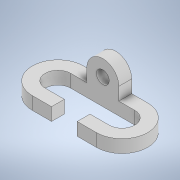
# Autodesk Inventor part: Assignment 3.4 - Coupling Base
Saved by Autodesk Inventor 2022 (Build 260153000, 153)
## iProperties
Created: 2021-05-23
Part Number: Assignment 3.4 - Coupling Base
Material: Generic
Document SubType Name: Modeling
Designer: Aaron
Density: 1 g/cm^3
Appearance: Default
Author: Aaron
Autodesk Inventor part; units mm, degrees
ref_plane "YZ Plane" through (0, 0, 0) normal (1, 0, 0) x (0, 1, 0)
ref_plane "XZ Plane" through (0, 0, 0) normal (0, 1, 0) x (-1, 0, 0)
ref_plane "XY Plane" through (0, 0, 0) normal (0, 0, 1) x (1, 0, 0)
sketch "Sketch1" plane through (0, 0, 0) normal (0, 1, 0) x (-1, 0, 0)
  line L0 (0, 0) -> (63.5, 0)
  arc A0 (63.5, 0) -> (63.5, 50.8) centre (63.5, 25.4) ccw
  arc A1 (63.5, 12.7) -> (63.5, 38.1) centre (63.5, 25.4) ccw
  line L1 (63.5, 12.7) -> (0, 12.7)
  arc A2 (0, 38.1) -> (0, 12.7) centre (0, 25.4) ccw
  arc A3 (0, 50.8) -> (0, 0) centre (0, 25.4) ccw
  line L2 (63.5, 38.1) -> (44.45, 38.1)
  line L3 (63.5, 50.8) -> (44.45, 50.8)
  line L4 (44.45, 50.8) -> (44.45, 38.1)
  line L5 (0, 50.8) -> (19.05, 50.8)
  line L6 (19.05, 50.8) -> (19.05, 38.1)
  line L7 (19.05, 38.1) -> (0, 38.1)
  point P0 (63.5, 50.8)
  dimension "d0" = 63.5
  dimension "d2" = 25.4
  dimension "d5" = 19.05
  dimension "d6" = 19.05
  constraints: 16 end point, 10 point on circle, 5 horizontal, 4 centre point, 3 perpendicular, 2 coincident
  measures "d0" distance of L0.end L0.start
  measures "d2" diameter of A1
  measures "d5" distance of L2.start L2.end
  measures "d6" distance of L5.start L5.end
extrude "Extrusion1" add sketch "Sketch1" against normal blind 12.7
sketch "Sketch2" plane through (-63.5, 0, 12.7) normal (0, 0, 1) x (1, 0, 0)
  line L0 (63.5, 0) -> (0, 0) projected
  line L1 (0, 0) -> (15.875, 0)
  line L2 (63.5, 0) -> (47.625, 0)
  line L3 (47.625, 0) -> (47.625, 12.7)
  line L4 (15.875, 0) -> (15.875, 12.7)
  circle A0 centre (31.75, 12.7) radius 6.35
  arc A1 (47.625, 12.7) -> (15.875, 12.7) centre (31.75, 12.7) ccw
  dimension "d9" = 15.875
  dimension "d10" = 15.875
  dimension "d11" = 12.7
  dimension "d12" = 12.7
  dimension "d15" = 12.7
  constraints: 8 end point, 2 centre point, 2 point on circle, 2 point on line, 1 coincident, 1 perpendicular, 1 vertical
  measures "d9" distance of L0.end L1.end
  measures "d10" distance of L0.start L2.end
  measures "d11" distance of L2.end L3.end
  measures "d12" distance of L1.end L4.end
  measures "d15" diameter of A0
extrude "Extrusion2" add sketch "Sketch2" against normal blind 12.7
body "Solid1"
